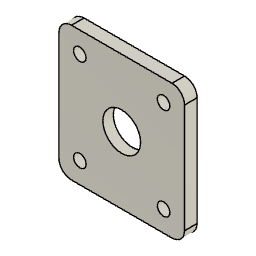
Magneto+Z+Spindel+Halter+oben+Teil1 (Autodesk Fusion 360 design; units mm, degrees)
Autodesk Fusion 360 part; units mm, degrees
note: some values were not read from the file. Chosen so that the rebuilt part matches the saved one: which face or edge a step refers to.
sketch "Skizze1" plane through (0, 0, 0) normal (0, 0, 1) x (1, 0, 0)
  line L0 (0, 0) -> (30, 0)
  line L1 (30, 0) -> (30, 30)
  line L2 (30, 30) -> (0, 30)
  line L3 (0, 30) -> (0, 0)
  circle A0 centre (15, 25) radius 2.1
  circle A1 centre (15, 5) radius 2.1
  line L4 (30, 20) -> (0, 20)
  line L5 (30, 10) -> (0, 10)
  dimension "d1" = 30
  dimension "d2" = 30
  dimension "d5" = 4.2
  dimension "d6" = 4.2
  constraint horizontal L0
  constraint vertical L1
  constraint horizontal L2
  constraint vertical L3
  constraint coincident L0.start L3.end
  measures "d1" distance of L0.start L0.end
  measures "d2" distance of L0.start L2.end
  measures "d5" diameter of A0
  measures "d6" diameter of A1
sketch "Skizze2" plane through (0, 10, 0) normal (0, -1, 0) x (1, 0, 0)
  line L0 (30, 0) -> (30, 46)
  line L1 (30, 46) -> (0, 46)
  line L2 (0, 46) -> (0, 0)
  circle A0 centre (15, 30) radius 11
  circle A1 centre (15, 30) radius 4.5
  line L3 (70, 14) -> (40, 14)
  line L4 (40, 14) -> (40, 46)
  line L5 (40, 46) -> (70, 46)
  line L6 (70, 46) -> (70, 14)
  circle A2 centre (55, 30) radius 4.5
  line L7 (40, 46) -> (45, 46)
  circle A3 centre (45, 41) radius 1.5
  circle A4 centre (65, 41) radius 1.5
  circle A5 centre (45, 19) radius 1.5
  circle A6 centre (65, 19) radius 1.5
  circle A7 centre (25, 41) radius 1.5
  circle A8 centre (5, 41) radius 1.5
  circle A9 centre (5, 19) radius 1.5
  circle A10 centre (25, 19) radius 1.5
  circle A11 centre (55, 30) radius 11
  line L8 (0, 0) -> (30, 0)
  point P0 (30, 0)
  dimension "d12" = 22
  dimension "d13" = 9
  dimension "d15" = 9
  dimension "d16" = 5
  dimension "d17" = 3
  dimension "d20" = 20
  dimension "d21" = -22
  dimension "d24" = 20
  dimension "d25" = -22
  dimension "d26" = 3
  dimension "d35" = 22
  constraint concentric A0 A1
  constraint horizontal L5
  constraint vertical L6
  constraint horizontal L3
  constraint vertical L4
  constraint coincident L5 L7.end
  constraint concentric A2 A11
  measures "d12" diameter of A0
  measures "d13" diameter of A1
  measures "d15" diameter of A2
  measures "d16" distance of L4.end L7.end
  measures "d17" diameter of A3
  measures "d26" diameter of A8
  measures "d35" diameter of A11
extrude "Extrusion6" add sketch "Skizze2" along normal blind 3 contours L3 L4 L5 L6 L7 | A11
extrude "Extrusion7" cut sketch "Skizze2" along normal blind 0.5 contours A11
fillet "Abrundung1" radius 3 4 edges at (70, 8.5, 14) (40, 8.5, 14) (70, 8.5, 46) (40, 8.5, 46)
